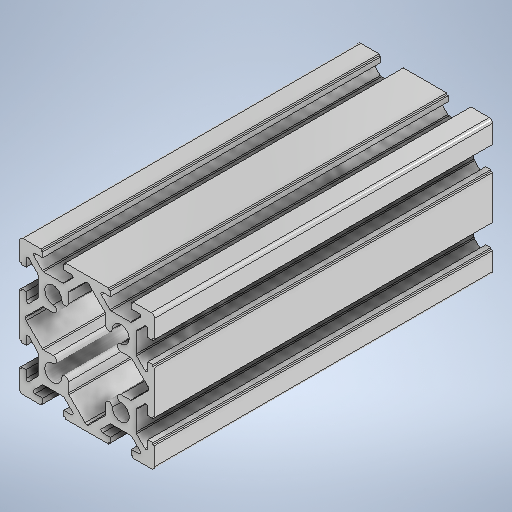
# Autodesk Inventor part: Perfil 40×40 8 rasgos_001
Saved by Autodesk Inventor 2026 (Build 300175000, 175)
## iProperties
Created: 2025-04-03
Part Number: Perfil 40×40 8 rasgos_001
Material: Aluminum 6061
Document SubType Name: Modeling
Designer: Carlos Dias
Density: 2.7 g/cm^3
Appearance: Aluminum - Polished
Author: Carlos Dias
Autodesk Inventor part; units mm, degrees
sketch "Sketch1" plane through (0, 0, 0) normal (0, 0, 1) x (1, 0, 0)
  line L0 (0, 20) -> (0, 0) construction
  line L1 (-20, 20) -> (0, 20) construction
  circle A0 centre (-10, 10) radius 2.5 construction
  line L2 (-14.5, 14.5) -> (-5.5, 14.5) construction
  line L3 (-5.5, 14.5) -> (-5.5, 5.5) construction
  line L4 (-14.5, 14.5) -> (-14.5, 5.5) construction
  line L5 (-14.5, 5.5) -> (-5.5, 5.5) construction
  line L6 (-1, 19) -> (-10, 10) construction
  line L7 (-19, 19) -> (-10, 10) construction
  line L8 (-19, 1) -> (-10, 10) construction
  line L9 (-3.4142, 18) -> (-6.9142, 14.5) construction
  line L10 (-0.5858, 18) -> (-5.5, 13.0858) construction
  line L11 (-6.9, 18) -> (-3.4142, 18) construction
  line L12 (-6.9, 20) -> (-6.9, 18) construction
  line L13 (-6.9, 20) -> (0, 20) construction
  line L14 (-16.5858, 18) -> (-13.0858, 14.5) construction
  line L15 (-18, 16.5858) -> (-14.5, 13.0858) construction
  line L16 (-20, 20) -> (-20, 0) construction
  line L17 (-16.5858, 18) -> (-13.1, 18) construction
  line L18 (-13.1, 20) -> (-13.1, 18) construction
  line L19 (-18, 16.5858) -> (-18, 13.1) construction
  line L20 (-18, 13.1) -> (-20, 13.1) construction
  line L21 (-13.0858, 5.5) -> (-18, 0.5858) construction
  line L22 (-14.5, 6.9142) -> (-18, 3.4142) construction
  line L23 (-18, 6.9) -> (-18, 3.4142) construction
  line L24 (-20, 6.9) -> (-18, 6.9) construction
  line L25 (-20, 13.1) -> (-19.5, 13.1) construction
  line L26 (-19.5, 13.1) -> (-19.5, 13.6)
  line L27 (-19.5, 13.6) -> (-20, 13.6)
  line L28 (-20, 13.6) -> (-20, 13.1) construction
  line L29 (-20, 6.9) -> (-19.5, 6.9) construction
  line L30 (-19.5, 6.9) -> (-19.5, 6.4)
  line L31 (-19.5, 6.4) -> (-20, 6.4)
  line L32 (-20, 6.4) -> (-20, 6.9) construction
  line L33 (-13.1, 20) -> (-13.6, 20) construction
  line L34 (-13.6, 20) -> (-13.6, 19.5)
  line L35 (-13.6, 19.5) -> (-13.1, 19.5)
  line L36 (-13.1, 19.5) -> (-13.1, 20) construction
  line L37 (-6.9, 20) -> (-6.4, 20) construction
  line L38 (-6.4, 20) -> (-6.4, 19.5)
  line L39 (-6.4, 19.5) -> (-6.9, 19.5)
  line L40 (-6.9, 19.5) -> (-6.9, 20) construction
  arc A1 (-19, 20) -> (-20, 19) centre (-19, 19) ccw
  arc A2 (-17.1464, 15.7322) -> (-18, 15.3787) centre (-17.5, 15.3787) ccw
  arc A3 (-14.5, 12.8787) -> (-14.6464, 13.2322) centre (-15, 12.8787) ccw
  arc A4 (-14.6464, 6.7678) -> (-14.5, 7.1213) centre (-15, 7.1213) ccw
  arc A5 (-18, 4.6213) -> (-17.1464, 4.2678) centre (-17.5, 4.6213) ccw
  arc A6 (-12.8787, 5.5) -> (-13.2322, 5.3536) centre (-12.8787, 5) ccw
  arc A7 (-15.3787, 18) -> (-15.7322, 17.1464) centre (-15.3787, 17.5) ccw
  arc A8 (-4.2678, 17.1464) -> (-4.6213, 18) centre (-4.6213, 17.5) ccw
  arc A9 (-13.2322, 14.6464) -> (-12.8787, 14.5) centre (-12.8787, 15) ccw
  arc A10 (-7.1213, 14.5) -> (-6.7678, 14.6464) centre (-7.1213, 15) ccw
  arc A11 (-5.3536, 13.2322) -> (-5.5, 12.8787) centre (-5, 12.8787) ccw
  arc A12 (0, 18.2855) -> (-0.5858, 18) centre (0.1213, 17.2929) ccw
  line L41 (0, 20) -> (0, 18.2855)
  line L42 (-6.4, 20) -> (0, 20)
  line L43 (-6.9, 19.5) -> (-6.9, 18)
  line L44 (-6.9, 18) -> (-4.6213, 18)
  line L45 (-4.2678, 17.1464) -> (-6.7678, 14.6464)
  line L46 (-0.5858, 18) -> (-5.3536, 13.2322)
  line L47 (-5.5, 12.8787) -> (-5.5, 10)
  line L48 (-12.8787, 14.5) -> (-7.1213, 14.5)
  line L49 (-12.8787, 5.5) -> (-10, 5.5)
  line L50 (-13.2322, 5.3536) -> (-18, 0.5858)
  line L51 (0, 0) -> (-20, 0) construction
  arc A13 (-18, 0.5858) -> (-18.2855, 0) centre (-17.2929, -0.1213) ccw
  line L52 (-14.6464, 6.7678) -> (-17.1464, 4.2678)
  line L53 (-20, 6.4) -> (-20, 0)
  line L54 (-20, 0) -> (-18.2855, 0)
  line L55 (-18, 6.9) -> (-18, 4.6213)
  line L56 (-18, 6.9) -> (-19.5, 6.9)
  line L57 (-14.5, 12.8787) -> (-14.5, 7.1213)
  line L58 (-17.1464, 15.7322) -> (-14.6464, 13.2322)
  line L59 (-18, 15.3787) -> (-18, 13.1)
  line L60 (-18, 13.1) -> (-19.5, 13.1)
  line L61 (-20, 19) -> (-20, 13.6)
  line L62 (-19, 20) -> (-13.6, 20)
  line L63 (-13.1, 19.5) -> (-13.1, 18)
  line L64 (-13.1, 18) -> (-15.3787, 18)
  line L65 (-15.7322, 17.1464) -> (-13.2322, 14.6464)
  arc A14 (-7.5, 10) -> (-10, 7.5) centre (-10, 10) ccw
  arc A15 (-10, 5.5) -> (-10, 7.5) centre (-10, 6.5) ccw
  arc A16 (-7.5, 10) -> (-5.5, 10) centre (-6.5, 10) ccw
  point P0 (-16.25, 14.8358)
  point P1 (-18, 5.1571)
  dimension "d3" = 5
  dimension "d0" = 20
  dimension "d1" = 20
  dimension "d4" = 10
  dimension "d5" = 10
  dimension "d6" = 2
  dimension "d8" = 2
  dimension "d9" = 4.5
  dimension "d10" = 4.5
  dimension "d11" = 1
  dimension "d12" = 2
  dimension "d13" = 1
  dimension "d14" = 3.1
  dimension "d15" = 1
  dimension "d16" = 1
  dimension "d17" = 2
  dimension "d18" = 3.1
  dimension "d19" = 1
  dimension "d20" = 1
  dimension "d21" = 0.5
  dimension "d23" = 1
  dimension "d24" = 0.5
  constraints: 132 end point, 35 point on line, 32 point on circle, 24 tangent, 17 horizontal, 16 centre point, 14 parallel, 13 equal length, 13 equal radius, 13 vertical, 7 midpoint, 6 horizontal alignment, 4 perpendicular, 3 vertical alignment, 2 coincident, 3 other
  measures "d0" distance of L0.start L0.end
  measures "d1" distance of L1.start L0.start
  measures "d4" horizontal distance of L0.start point (-10, 10)
  measures "d5" horizontal distance of point (0, 0) point (-10, 10)
  measures "d9" distance from line of L4 point (-10, 10)
  measures "d10" distance of A15.start point (-10, 10)
  measures "d11" distance between parallel lines of L6 L9
  measures "d12" distance from line of L1 L9.start
  measures "d13" distance between parallel lines of L10 L6
  measures "d14" horizontal distance of point (-10, 10) L11.start
  measures "d15" distance between parallel lines of L7 L14
  measures "d16" distance from line of L7 point (-16.25, 14.836)
  measures "d17" distance from line of L16 L15.start
  measures "d18" horizontal distance of L6.end L17.end
  measures "d19" distance between parallel lines of L8 L21
  measures "d20" distance between parallel lines of L8 L22
  measures "d21" distance of L26.end L27.end
  measures "d23" radius of A1
  measures "d24" radius of A2
extrude "Extrusion1" add sketch "Sketch1" along normal mid plane 100
mirror "Mirror1" about plane through (0, 0, 0) normal (0, 1, 0) of "Extrusion1"
mirror "Mirror2" about plane through (0, 0, 0) normal (1, 0, 0) of "Extrusion1", "Mirror1"
equation "\"d8\" = d6"
equation "\"d13\" = d11"
equation "\"d15\" = d11"
equation "\"d16\" = d11"
equation "\"d19\" = d11"
equation "\"d20\" = d11"
body "Solid1"
